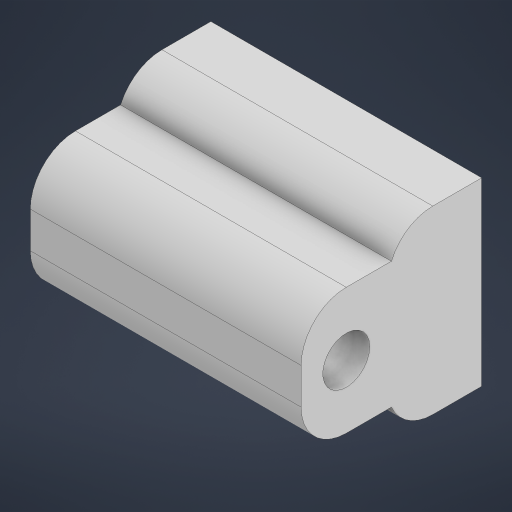
# Autodesk Inventor part: Torsion_Spring_Mounts
Saved by Autodesk Inventor 2023 (Build 270158000, 158)
## iProperties
Created: 2024-02-21
Part Number: Torsion_Spring_Mounts
Material: Generic
Document SubType Name: Modeling
Designer: kelle
Density: 1 g/cm^3
Appearance: Default
Author: kelle
Autodesk Inventor part; units mm, degrees
ref_plane "YZ Plane" through (0, 0, 0) normal (1, 0, 0) x (0, 1, 0)
ref_plane "XZ Plane" through (0, 0, 0) normal (0, 1, 0) x (-1, 0, 0)
ref_plane "XY Plane" through (0, 0, 0) normal (0, 0, 1) x (1, 0, 0)
sketch "Sketch1" plane through (0, 0, 0) normal (0, 0, 1) x (1, 0, 0)
  line L0 (9.525, -6.35) -> (-9.525, -6.35)
  line L1 (-9.525, -6.35) -> (-9.525, 6.35)
  line L2 (-9.525, 6.35) -> (9.525, 6.35)
  line L3 (9.525, 6.35) -> (9.525, -6.35)
  line L4 (9.525, -6.35) -> (-9.525, 6.35) construction
  line L5 (-9.525, -6.35) -> (9.525, 6.35) construction
  point P0 (0, 0)
  dimension "d0" = 19.05
  dimension "d1" = 12.7
  constraints: 12 end point, 2 midpoint, 2 parallel, 1 horizontal, 1 perpendicular
  measures "d0" distance of L1.end L2.end
  measures "d1" distance of L0.end L1.end
extrude "Extrusion1" add sketch "Sketch1" along normal blind 6.35
sketch "Sketch2" plane through (0, 0, 6.35) normal (0, 0, 1) x (1, 0, 0)
  line L0 (9.525, 6.35) -> (-9.525, 6.35) projected
  line L1 (-9.525, 6.35) -> (-9.525, -6.35) projected
  line L2 (-9.525, -6.35) -> (9.525, -6.35) projected
  line L3 (9.525, -6.35) -> (9.525, 6.35) projected
  line L4 (9.525, -4.445) -> (-9.525, -4.445)
  line L5 (-9.525, -4.445) -> (-9.525, 4.445)
  line L6 (-9.525, 4.445) -> (9.525, 4.445)
  line L7 (9.525, 4.445) -> (9.525, -4.445)
  line L8 (9.525, -4.445) -> (-9.525, 4.445) construction
  line L9 (-9.525, -4.445) -> (9.525, 4.445) construction
  point P0 (0, 0)
  dimension "d4" = 19.05
  dimension "d5" = 8.89
  constraints: 12 end point, 2 midpoint, 2 parallel, 1 horizontal, 1 perpendicular
  measures "d4" distance of L5.end L6.end
  measures "d5" distance of L4.end L5.end
extrude "Extrusion2" add sketch "Sketch2" along normal blind 6.35 contours L3 L4 L1 L6
sketch "Sketch3" plane through (9.525, -6.35, 0) normal (1, 0, 0) x (0, 0, -1)
  line L0 (0, 0) -> (0, 12.7) projected
  line L1 (0, 12.7) -> (-6.35, 12.7) projected
  line L2 (-6.35, 10.795) -> (-6.35, 12.7) projected
  line L3 (-6.35, 10.795) -> (-12.7, 10.795) projected
  line L4 (-12.7, 1.905) -> (-12.7, 10.795) projected
  line L5 (-6.35, 1.905) -> (-12.7, 1.905) projected
  line L6 (-6.35, 0) -> (-6.35, 1.905) projected
  line L7 (0, 0) -> (-6.35, 0) projected
  line L8 (-6.35, 12.7) -> (-6.35, 10.795) construction
  line L9 (-6.35, 10.795) -> (-6.35, 1.905) construction
  line L10 (-12.7, 6.35) -> (0, 6.35) construction
  line L11 (-9.525, 10.795) -> (-9.525, 1.905) construction
  line L12 (-6.35, 1.905) -> (-12.7, 1.905) construction
  circle A0 centre (-9.525, 6.35) radius 1.651
  dimension "d8" = 3.302
  constraints: 6 end point, 4 midpoint, 1 centre point, 1 collinear, 1 horizontal
  measures "d8" diameter of A0
extrude "Extrusion3" cut sketch "Sketch3" against normal through all contours A0
fillet "Fillet1" radius 3.175 4 edges at (0, 4.445, 12.7) (0, -4.445, 12.7) (0, 6.35, 6.35) (0, -6.35, 6.35)
body "Solid1"
